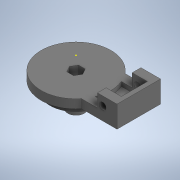
# Autodesk Inventor part: celestronTripodAdapterTop
Saved by Autodesk Inventor 2021.1 (Build 251245000, 245)
## iProperties
Created: 2020-07-29
Part Number: celestronTripodAdapterTop
Material: PC/ABS Plastic
Document SubType Name: Modeling
Designer: robst
Density: 0.357273 g/cm^3
Appearance: Gray
Author: robst
Autodesk Inventor part; units mm, degrees
ref_plane "YZ Plane" through (0, 0, 0) normal (1, 0, 0) x (0, 1, 0)
ref_plane "XZ Plane" through (0, 0, 0) normal (0, 1, 0) x (-1, 0, 0)
ref_plane "XY Plane" through (0, 0, 0) normal (0, 0, 1) x (1, 0, 0)
sketch "Sketch1" plane through (0, 0, 0) normal (0, 0, 1) x (1, 0, 0)
  line L0 (0, 0) -> (-50.8, 0)
  line L1 (-50.8, 0) -> (-50.8, -12.7)
  line L2 (-50.8, -12.7) -> (-38.1, -12.7)
  line L3 (-12.0663, -25.4) -> (-12.0663, -48.26)
  line L4 (-5, -48.26) -> (-5, -16.764)
  line L5 (-5, -16.764) -> (0, -16.764)
  line L6 (0, -16.764) -> (0, 0)
  line L7 (-12.0663, -48.26) -> (-5, -48.26)
  line L8 (-38.1, -12.7) -> (-38.1, -25.4)
  line L9 (-38.1, -25.4) -> (-12.0663, -25.4)
  dimension "d0" = 50.8
  dimension "d1" = 5
  dimension "d2" = 12.0663
  dimension "d13" = 35.56
  dimension "d15" = 31.496
  dimension "d38" = 12.7
  dimension "d39" = 38.1
  constraints: 20 end point, 7 perpendicular, 1 horizontal, 1 vertical
  measures "d0" distance of L0.end L0.start
  measures "d1" distance of L5.end L4.end
  measures "d2" distance from line of L3 L0.start
  measures "d13" distance between parallel lines of L7 L2
  measures "d15" vertical distance of L4.start L5.end
  measures "d38" distance between parallel lines of L9 L2
  measures "d39" distance from line of L8 L0.start
revolve "Revolution1" add sketch "Sketch1" angle 360 about axis through (0, -16.764, 0) along (0, 1, 0)
sketch "Sketch5" plane through (0, 0, 0) normal (0, 1, 0) x (1, 0, 0)
  circle A0 centre (0, 0) radius 5 projected
  line L0 (9.815, 0) -> (4.9075, -8.5)
  line L1 (4.9075, -8.5) -> (-4.9075, -8.5)
  line L2 (-4.9075, -8.5) -> (-9.815, 0)
  line L3 (-9.815, 0) -> (-4.9075, 8.5)
  line L4 (-4.9075, 8.5) -> (4.9075, 8.5)
  line L5 (4.9075, 8.5) -> (9.815, 0)
  point P0 (0, 0)
  point P1 (0, 0)
  dimension "d16" = 17
  constraints: 12 end point, 1 coincident, 1 horizontal, 13 other
  measures "d16" distance between parallel lines of L3 L0
extrude "Extrusion1" cut sketch "Sketch5" against normal blind 12.7 contours A0 | L0 L1 L2 L3 L4 L5
sketch "Sketch7" plane through (0, -12.7, 0) normal (0, -1, 0) x (1, 0, 0)
  circle A0 centre (0, 0) radius 50.8 projected
  line L0 (47.0929, -19.05) -> (85.1929, -19.05)
  line L1 (85.1929, -19.05) -> (85.1929, -31.75)
  line L2 (85.1929, -31.75) -> (39.6557, -31.75)
  circle A1 centre (0, 0) radius 5 construction
  line L3 (0, 0) -> (5, 0) construction
  line L4 (50.8, 0) -> (83.823, 0) construction
  dimension "d23" = 38.1
  dimension "d24" = 12.7
  dimension "d25" = 19.05
  constraints: 10 end point, 3 horizontal, 3 point on circle, 2 perpendicular, 1 horizontal alignment, 1 other
  measures "d23" distance of L0.start L0.end
  measures "d24" distance of L0.end L1.end
  measures "d25" distance from line of L0 point (0, 0)
extrude "Extrusion3" add sketch "Sketch7" against normal blind 12.7 contours A0 L0 L1 L2
sketch "Sketch8" plane through (39.6557, 0, -31.75) normal (0, 1, 0) x (1, 0, 0)
  line L0 (45.5371, -12.7) -> (45.5371, 0) projected
  line L1 (45.5371, 0) -> (0, 0) projected
  line L2 (7.4371, -12.7) -> (45.5371, -12.7) projected
  line L3 (35.8511, -107.95) -> (35.8511, 44.45)
  line L4 (26.3261, -107.95) -> (26.3261, 44.45)
  line L5 (45.5371, -12.7) -> (23.3121, -12.7)
  line L6 (23.3121, -12.7) -> (23.3121, 0)
  line L7 (23.3121, 0) -> (45.5371, 0)
  line L8 (45.5371, 0) -> (45.5371, -12.7)
  point P0 (-39.6557, -31.75)
  point P1 (23.3121, 0)
  point P2 (23.3121, -12.7)
  dimension "d28" = 22.225
  constraints: 12 end point, 2 parallel, 2 vertical, 1 collinear, 1 horizontal, 1 perpendicular, 4 other
  measures "d28" distance of L6.end L7.end
extrude "Extrusion4" add sketch "Sketch8" along normal blind 19.05
sketch "Sketch9" plane through (85.1929, -12.7, -31.75) normal (0, 0, -1) x (-1, 0, 0)
  line L0 (22.225, 12.7) -> (22.225, 31.75) projected
  line L1 (0, 31.75) -> (22.225, 31.75) projected
  arc A0 (16.0423, 14.3621) -> (12.8546, 14.3621) centre (14.4485, 18.85) ccw projected
  line L2 (0, 0) -> (0, 31.75) projected
  circle A1 centre (14.4485, 18.85) radius 4.953
  point P0 (85.1929, 12.7)
  dimension "d31" = 9.906
  constraints: 1 centre point, 1 coincident
  measures "d31" diameter of A1
extrude "Extrusion5" cut sketch "Sketch9" against normal through all
mirror "Mirror1" about plane through (0, 0, 0) normal (0, 0, 1) of "Extrusion4", "Extrusion5", "Extrusion3"
sketch "Sketch10" plane through (39.6557, -12.7, -31.75) normal (0, -1, 0) x (1, 0, 0)
  arc A0 (7.4371, 12.7) -> (7.4371, 50.8) centre (-39.6557, 31.75) ccw projected
  line L0 (45.5371, 50.8) -> (7.4371, 50.8) projected
  line L1 (45.5371, 12.7) -> (7.4371, 12.7) projected
  arc A1 (7.4371, 12.7) -> (7.4371, 50.8) centre (-39.6557, 31.75) ccw
  line L2 (7.4371, 50.8) -> (45.5371, 50.8)
  line L3 (45.5371, 0) -> (45.5371, 12.7) projected
  line L4 (45.5371, 50.8) -> (45.5371, 12.7)
  line L5 (45.5371, 12.7) -> (7.4371, 12.7)
  constraints: 7 end point, 2 collinear, 2 point on circle, 1 centre point, 1 coincident, 1 perpendicular
extrude "Extrusion6" add sketch "Sketch10" against normal blind 6.35
sketch "Sketch11" plane through (85.1929, -12.7, -31.75) normal (1, 0, 0) x (0, 0, -1)
  line L0 (-63.5, 0) -> (-63.5, 31.75) projected
  line L1 (-50.8, 31.75) -> (-63.5, 31.75) projected
  line L2 (-12.7, 31.75) -> (0, 31.75) projected
  line L3 (0, 0) -> (0, 31.75) projected
  line L4 (0, 0) -> (-63.5, 0) projected
  line L5 (-63.5, 31.75) -> (0, 31.75)
  line L6 (0, 31.75) -> (0, 0)
  line L7 (0, 0) -> (-63.5, 0)
  line L8 (-63.5, 0) -> (-63.5, 31.75)
  point P0 (-31.75, 12.7)
  point P1 (-12.7, 31.75)
  point P2 (-50.8, 31.75)
  constraints: 8 end point, 2 parallel, 1 horizontal, 1 perpendicular
extrude "Extrusion7" add sketch "Sketch11" along normal blind 6.35
sketch "Sketch12" plane through (39.6557, 19.05, -31.75) normal (0, 1, 0) x (1, 0, 0)
  point P0 (-39.6557, -31.75)
equation "\"d0\" = topPartRadius"
equation "\"d2\" = stemRadius"
equation "\"d15\" = internalHoleDepth"
equation "\"topPartRadius\" = 0.5 * topPartDiameter"
equation "\"totalHeight\" = 35.56"
equation "\"stemRadius\" = 12.06627"
equation "\"stemHeight\" = 22.86"
equation "\"internalHoleDepth\" = 31.496"
equation "\"topPartDiameter\" = 101.6"
body "Solid1"
